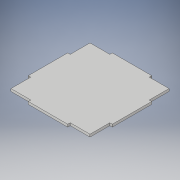
# Autodesk Inventor part: BASE_FONDO
Saved by Autodesk Inventor 2019 (Build 230136000, 136)
## iProperties
Created: 2020-02-12
Part Number: BASE_FONDO
Material: Genérico
Document SubType Name: Modeling
Designer: omar-
Density: 1 g/cm^3
Appearance: Valor por defecto
Author: omar-
Autodesk Inventor part; units mm, degrees
ref_plane "YZ Plane" through (0, 0, 0) normal (1, 0, 0) x (0, 1, 0)
ref_plane "XZ Plane" through (0, 0, 0) normal (0, 1, 0) x (-1, 0, 0)
ref_plane "XY Plane" through (0, 0, 0) normal (0, 0, 1) x (1, 0, 0)
sketch "Boceto1" plane through (0, 0, 0) normal (0, 1, 0) x (-1, 0, 0)
  line L0 (-50, 50) -> (50, 50)
  line L1 (50, 50) -> (50, -50)
  line L2 (50, -50) -> (-50, -50)
  line L3 (-50, -50) -> (-50, 50)
  line L4 (-50, 50) -> (50, -50) construction
  line L5 (50, 50) -> (-50, -50) construction
  line L6 (25, 53.18) -> (-25, 53.18)
  line L7 (-25, 53.18) -> (-25, 50)
  line L8 (-25, 50) -> (25, 50)
  line L9 (25, 50) -> (25, 53.18)
  line L10 (25, -50) -> (-25, -50)
  line L11 (-25, -50) -> (-25, -53.18)
  line L12 (-25, -53.18) -> (25, -53.18)
  line L13 (25, -53.18) -> (25, -50)
  line L14 (53.18, 25) -> (50, 25)
  line L15 (50, 25) -> (50, -25)
  line L16 (50, -25) -> (53.18, -25)
  line L17 (53.18, -25) -> (53.18, 25)
  line L18 (-50, 25) -> (-53.18, 25)
  line L19 (-53.18, 25) -> (-53.18, -25)
  line L20 (-53.18, -25) -> (-50, -25)
  line L21 (-50, -25) -> (-50, 25)
  point P0 (0, 0)
  dimension "d0" = 100
  dimension "d1" = 100
  dimension "d2" = 3.18
  dimension "d3" = 3.18
  dimension "d4" = 50
  dimension "d5" = 25
  dimension "d6" = 25
  dimension "d7" = 25
  constraints: 44 end point, 10 parallel, 9 perpendicular, 5 collinear, 5 horizontal, 2 midpoint, 1 point on line
  measures "d0" distance of L1.end L2.end
  measures "d1" distance of L0.end L1.end
  measures "d2" distance of L12.end L10.start
  measures "d3" distance of L8.end L6.start
  measures "d4" distance of L11.end L12.end
  measures "d5" distance between parallel lines of L1 L13
  measures "d6" distance between parallel lines of L1 L9
  measures "d7" distance between parallel lines of L2 L16
extrude "Extrusión1" add sketch "Boceto1" along normal blind 3.18
